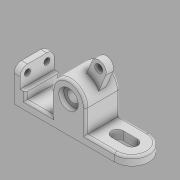
# Autodesk Inventor part: Support A01209499
Saved by Autodesk Inventor 2020 (Build 240168000, 168)
## iProperties
Created: 2019-09-18
Part Number: Support A01209499
Material: Genérico
Document SubType Name: Modeling
Designer: gerar
Density: 1 g/cm^3
Appearance: Valor por defecto
Author: gerar
Autodesk Inventor part; units mm, degrees
ref_plane "YZ Plane" through (0, 0, 0) normal (1, 0, 0) x (0, 1, 0)
ref_plane "XZ Plane" through (0, 0, 0) normal (0, 1, 0) x (-1, 0, 0)
ref_plane "XY Plane" through (0, 0, 0) normal (0, 0, 1) x (1, 0, 0)
sketch "Boceto1" plane through (0, 0, 0) normal (0, 0, 1) x (1, 0, 0)
  line L0 (0, 0) -> (7.874, 0)
  line L1 (7.874, 0) -> (7.874, 44.45)
  line L2 (7.874, 44.45) -> (0, 44.45)
  line L3 (0, 44.45) -> (0, 0)
  line L4 (7.874, 0) -> (14.986, 0)
  line L5 (14.986, 0) -> (14.986, 20.574)
  line L6 (14.986, 20.574) -> (7.874, 20.574)
  line L7 (7.874, 20.574) -> (7.874, 0)
  line L8 (14.986, 0) -> (154.178, 0)
  line L9 (154.178, 0) -> (154.178, 11.176)
  line L10 (154.178, 11.176) -> (14.986, 11.176)
  line L11 (14.986, 11.176) -> (14.986, 0)
  line L12 (71.374, -17.734) -> (71.374, 53.7608) construction
  line L13 (-9.4803, 41.148) -> (163.4374, 41.148) construction
  arc A0 (93.726, 41.148) -> (49.022, 41.148) centre (71.374, 41.148) ccw
  line L14 (49.022, 41.148) -> (49.022, 11.176)
  line L15 (93.726, 41.148) -> (93.726, 11.176)
  point P0 (14.986, 11.176)
  dimension "d0" = 7.874
  dimension "d1" = 44.45
  dimension "d2" = 7.112
  dimension "d3" = 20.574
  dimension "d4" = 139.192
  dimension "d5" = 11.176
  dimension "d6" = 63.5
  dimension "d7" = 41.148
  dimension "d8" = 44.704
  constraints: 32 end point, 6 parallel, 6 point on line, 5 perpendicular, 4 horizontal, 2 point on circle, 2 tangent, 1 centre point, 1 vertical
  measures "d0" distance of L2.end L1.end
  measures "d1" distance between parallel lines of L0 L2
  measures "d2" distance of L6.end L5.end
  measures "d3" distance of L5.end L4.end
  measures "d4" distance of L10.end L9.end
  measures "d5" distance between parallel lines of L8 L10
  measures "d6" distance between parallel lines of L1 L12
  measures "d7" distance between parallel lines of L8 L13
  measures "d8" diameter of A0
extrude "Base" add sketch "Boceto1" against normal blind 44.704
sketch "Boceto2" plane through (0, 0, 0) normal (-1, 0, 0) x (0, 0, 1)
  line L0 (0, 44.45) -> (-44.704, 44.45) projected
  line L1 (-35.052, 44.45) -> (-9.652, 44.45)
  line L2 (0, 34.798) -> (0, 0)
  line L3 (0, 0) -> (-44.704, 0)
  line L4 (-44.704, 0) -> (-44.704, 34.798)
  arc A0 (-35.052, 44.45) -> (-44.704, 34.798) centre (-35.052, 34.798) ccw
  arc A1 (0, 34.798) -> (-9.652, 44.45) centre (-9.652, 34.798) ccw
  line L5 (-44.704, 34.798) -> (-44.704, 44.45)
  line L6 (-44.704, 41.148) -> (-44.704, 11.176) projected
  line L7 (-44.704, 44.45) -> (-35.052, 44.45)
  line L8 (-9.652, 44.45) -> (0, 44.45)
  line L9 (0, 44.45) -> (0, 34.798)
  line L10 (0, 11.176) -> (0, 41.148) projected
  arc A2 (-35.052, 44.45) -> (-41.877, 41.623) centre (-35.052, 34.798) ccw
  arc A3 (0, 34.798) -> (-2.827, 41.623) centre (-9.652, 34.798) ccw
  dimension "d11" = 9.652
  constraints: 16 end point, 13 point on circle, 7 tangent, 5 point on line, 4 centre point, 2 collinear, 2 parallel, 1 equal radius, 1 horizontal, 1 perpendicular
  measures "d11" radius of A0
extrude "RedondeoIzquierda" cut sketch "Boceto2" against normal blind 7.874 contours L9 A1 L0 | A0 L5 L0
sketch "Boceto3" plane through (93.726, 11.176, 0) normal (0, 1, 0) x (1, 0, 0)
  line L0 (38.1, 57.3464) -> (38.1, -17.2234) construction
  line L1 (80.6333, 22.352) -> (-7.9842, 22.352) construction
  line L2 (60.452, 0) -> (60.452, 44.704) projected
  line L3 (60.452, 0) -> (0, 0) projected
  line L4 (0, 44.704) -> (60.452, 44.704) projected
  line L5 (-22.352, 117.0356) -> (-22.352, -54.5943) construction
  arc A0 (38.1, 0) -> (38.1, 44.704) centre (38.1, 22.352) ccw
  point P0 (-93.726, 0)
  point P1 (60.452, 22.352)
  dimension "d14" = 22.352
  dimension "d15" = 44.704
  dimension "d16" = 22.352
  dimension "d17" = 71.374
  dimension "d18" = 60.452
  dimension "d19" = 44.704
  constraints: 6 end point, 4 point on line, 2 point on circle, 2 vertical, 1 centre point, 1 horizontal
  measures "d14" distance between parallel lines of L0 L2
  measures "d15" distance between parallel lines of L3 L4
  measures "d16" distance between parallel lines of L4 L1
  measures "d17" distance from line of point (-93.726, 0) L5
  measures "d18" distance between parallel lines of L0 L5
  measures "d19" diameter of A0
extrude "RedondeoDerecha" cut sketch "Boceto3" against normal blind 11.176
sketch "Boceto4" plane through (93.726, 11.176, 0) normal (0, 1, 0) x (1, 0, 0)
  line L0 (53.4052, 29.8958) -> (-6.9452, 29.8958) construction
  line L1 (53.4052, 14.8082) -> (-2.7405, 14.8082) construction
  line L2 (0, 44.704) -> (38.1, 44.704) projected
  line L3 (38.1, 0) -> (0, 0) projected
  line L4 (40.7958, 60.876) -> (40.7958, -13.6937) construction
  arc A0 (38.1, 0) -> (38.1, 44.704) centre (38.1, 22.352) ccw construction
  arc A1 (38.1, 14.8082) -> (38.1, 29.8958) centre (38.1, 22.352) ccw
  line L5 (38.1, 22.352) -> (19.05, 22.352) construction
  arc A2 (19.05, 29.8958) -> (19.05, 14.8082) centre (19.05, 22.352) ccw
  line L6 (19.05, 29.8958) -> (38.1, 29.8958)
  line L7 (19.05, 14.8082) -> (38.1, 14.8082)
  point P0 (-93.726, 0)
  dimension "d22" = 15.0876
  dimension "d23" = 44.704
  dimension "d24" = 14.8082
  dimension "d26" = 19.05
  constraints: 12 end point, 4 parallel, 4 point on circle, 4 point on line, 3 horizontal, 2 centre point, 2 coincident, 2 tangent, 1 vertical
  measures "d22" distance between parallel lines of L1 L0
  measures "d23" distance between parallel lines of L3 L2
  measures "d24" distance between parallel lines of L0 L2
  measures "d26" distance of L5.start L5.end
extrude "HuecoDerecha" cut sketch "Boceto4" against normal blind 11.176
sketch "Boceto5" plane through (0, 0, 0) normal (0, 0, 1) x (1, 0, 0)
  arc A0 (93.726, 41.148) -> (49.022, 41.148) centre (71.374, 41.148) ccw construction
  point P0 (0, 0)
  constraints: 1 coincident
hole "AgujeroCentral" at (71.374, 41.148, 0) direction (0, 0, -1) diameter 15.4686 end through all counterbore diameter 25.4 counterbore depth 6.35
sketch "Boceto6" plane through (0, 0, -44.704) normal (-1, 0, 0) x (0, 0, 1)
  arc A0 (44.704, 34.798) -> (35.052, 44.45) centre (35.052, 34.798) ccw projected
  arc A1 (9.652, 44.45) -> (0, 34.798) centre (9.652, 34.798) ccw projected
  circle A2 centre (9.652, 34.798) radius 3.9624
  circle A3 centre (35.052, 34.798) radius 3.9624
  line L0 (0, 0) -> (0, 34.798) projected
  line L1 (44.704, 34.798) -> (44.704, 0) projected
  line L2 (35.052, 44.45) -> (9.652, 44.45) projected
  line L3 (44.704, 0) -> (0, 0) projected
  dimension "d36" = 7.9248
  dimension "d37" = 7.9248
  dimension "d38" = 9.652
  dimension "d39" = 9.652
  dimension "d40" = 9.652
  dimension "d41" = 9.652
  dimension "d42" = 34.798
  dimension "d43" = 25.4
  constraints: 2 centre point, 2 coincident
  measures "d36" diameter of A2
  measures "d37" diameter of A3
  measures "d38" distance from line of L0 A1.centre
  measures "d39" distance from line of L1 A0.centre
  measures "d40" distance from line of A1.centre L2
  measures "d41" distance from line of L2 A0.centre
  measures "d42" distance from line of L3 A1.centre
  measures "d43" distance of A0.centre A1.centre
extrude "HuecosIzquierda" cut sketch "Boceto6" against normal blind 7.874 contours A2 | A3
sketch "Boceto7" plane through (0, 0, 0) normal (0, 0, 1) x (1, 0, 0)
  arc A0 (93.726, 41.148) -> (49.022, 41.148) centre (71.374, 41.148) ccw projected
  line L0 (93.726, 11.176) -> (93.726, 41.148) construction
  line L1 (49.022, 11.176) -> (14.986, 11.176) construction
  line L2 (93.726, 11.176) -> (49.022, 11.176) construction
  line L3 (71.374, 11.176) -> (71.374, 79.2986) construction
  line L4 (71.374, 11.176) -> (150.9411, 11.176) construction
  line L5 (71.374, 41.148) -> (130.1866, 41.148) construction
  line L6 (71.374, 41.148) -> (127.2183, 41.148) construction
  arc A1 (93.726, 41.148) -> (49.022, 41.148) centre (71.374, 41.148) ccw construction
  arc A2 (93.726, 41.148) -> (49.022, 41.148) centre (71.374, 41.148) ccw construction
  line L7 (93.726, 11.176) -> (93.726, 41.148) construction
  line L8 (93.726, 41.148) -> (93.726, 11.176) construction
  line L9 (71.374, 41.148) -> (91.948, 76.7832) construction
  line L10 (71.374, 41.148) -> (112.522, 41.148) construction
  arc A3 (100.8759, 73.1152) -> (83.0201, 80.4513) centre (91.948, 76.7832) ccw
  arc A4 (93.726, 41.148) -> (49.022, 41.148) centre (71.374, 41.148) ccw projected
  line L11 (75.8681, 63.0435) -> (83.0201, 80.4513)
  line L12 (91.6272, 50.6043) -> (100.8759, 73.1152)
  point P0 (0, 0)
  dimension "d48" = 22.352
  dimension "d49" = 41.148
  dimension "d50" = 60
  dimension "d51" = 19.304
  constraints: 18 end point, 5 horizontal, 3 point on circle, 2 tangent, 1 centre point, 1 coincident, 1 equal length, 1 midpoint, 1 parallel, 1 vertical, 2 other
  measures "d48" radius of A0
  measures "d49" distance of L9.start L9.end
  measures "d50" angle of L10 L9
  measures "d51" diameter of A3
extrude "Protuberancia" add sketch "Boceto7" against normal blind 44.704 separate body
sketch "Boceto8" plane through (0, 0, 0) normal (0, 0, 1) x (1, 0, 0)
  arc A0 (100.8759, 73.1152) -> (83.0201, 80.4513) centre (91.948, 76.7832) ccw projected
  arc A1 (100.8759, 73.1152) -> (83.0201, 80.4513) centre (91.948, 76.7832) ccw
  line L0 (75.8681, 63.0435) -> (83.0201, 80.4513) projected
  line L1 (83.0201, 80.4513) -> (75.8681, 63.0435)
  line L2 (100.8759, 73.1152) -> (91.6272, 50.6043) projected
  line L3 (100.8759, 73.1152) -> (91.6272, 50.6043)
  arc A2 (93.726, 41.148) -> (49.022, 41.148) centre (71.374, 41.148) ccw projected
  arc A3 (91.6272, 50.6043) -> (75.8681, 63.0435) centre (71.374, 41.148) ccw
  point P0 (0, 0)
  constraints: 4 end point, 4 point on circle, 2 centre point, 2 coincident, 2 collinear, 1 tangent
extrude "RestoFrontalProtuberancia" cut sketch "Boceto8" against normal blind 19.05 bodies 2
sketch "Boceto9" plane through (0, 0, -44.704) normal (0, 0, -1) x (-1, 0, 0)
  arc A0 (-49.022, 41.148) -> (-93.726, 41.148) centre (-71.374, 41.148) ccw projected
  arc A1 (-83.0201, 80.4513) -> (-100.8759, 73.1152) centre (-91.948, 76.7832) ccw projected
  line L0 (-100.8759, 73.1152) -> (-91.6272, 50.6043) projected
  line L1 (-75.8681, 63.0435) -> (-83.0201, 80.4513) projected
  point P0 (0, 0)
extrude "RestoTraseroProtuberancia" cut sketch "Boceto9" against normal blind 16.002 bodies 2
sketch "Boceto10" plane through (0, 0, -19.05) normal (0, 0, 1) x (1, 0, 0)
  arc A0 (100.8759, 73.1152) -> (83.0201, 80.4513) centre (91.948, 76.7832) ccw projected
  circle A1 centre (91.948, 76.7832) radius 5.1562
  point P0 (0, 0)
  dimension "d58" = 10.3124
  constraints: 1 centre point, 1 coincident
  measures "d58" diameter of A1
extrude "HuecoProtuberancia" cut sketch "Boceto10" against normal blind 9.652 bodies 2
fillet "Empalmes" radius 3.048 13 edges at (14.986, 15.875, 0) (32.004, 11.176, 0) (71.374, 63.5, 0) (93.726, 26.162, 0) (49.022, 26.162, 0) (154.178, 11.176, -22.352) (112.776, 11.176, -44.704) (112.776, 11.176, 0) (71.374, 63.5, -44.704) (49.022, 26.162, -44.704) (93.726, 26.162, -44.704) (32.004, 11.176, -44.704) (14.986, 15.875, -44.704)
equation "\"d16\" = 0.5 * d15"
equation "\"d24\" = -0.5 * d22 + 0.5 * d23"
